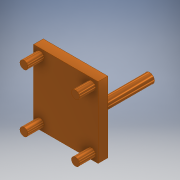
# Autodesk Inventor part: slider
Saved by Autodesk Inventor 2018 (Build 220112000, 112)
## iProperties
Created: 2024-05-02
Part Number: slider
Material: Gold
Document SubType Name: Modeling
Designer: neo
Density: 19.3 g/cm^3
Appearance: Metal 1600F Hot
Author: neo
Autodesk Inventor part; units mm, degrees
ref_plane "YZ Plane" through (0, 0, 0) normal (1, 0, 0) x (0, 1, 0)
ref_plane "XZ Plane" through (0, 0, 0) normal (0, 1, 0) x (-1, 0, 0)
ref_plane "XY Plane" through (0, 0, 0) normal (0, 0, 1) x (1, 0, 0)
sketch "Sketch1" plane through (0, 0, 0) normal (0, 1, 0) x (-1, 0, 0)
  line L0 (15.7413, 3.3999) -> (-17.2771, 3.3999)
  line L1 (0.4016, 18.4289) -> (0.4016, -19.5807)
  line L2 (10.4016, 14.3999) -> (-9.5984, 14.3999)
  line L3 (-9.5984, 14.3999) -> (-9.5984, -7.6001)
  line L4 (-9.5984, -7.6001) -> (10.4016, -7.6001)
  line L5 (10.4016, -7.6001) -> (10.4016, 14.3999)
  circle A0 centre (8.4016, 12.3999) radius 1.25
  circle A1 centre (8.4016, -5.6001) radius 1.25
  circle A2 centre (-7.5984, 12.3999) radius 1.25
  circle A3 centre (-7.5984, -5.6001) radius 1.25
  circle A4 centre (-5.5984, 3.3999) radius 1.5
  point P0 (0, 0)
  dimension "d0" = 2.5
  dimension "d1" = 18
  dimension "d2" = 22
  dimension "d3" = 20
  dimension "d4" = 16
  dimension "d5" = 3
  dimension "d6" = 16
  constraints: 12 end point, 5 centre point, 3 symmetric about line, 2 horizontal, 2 parallel, 1 perpendicular, 1 point on line, 1 vertical, 5 other
  measures "d0" diameter of A0
  measures "d1" distance of A1.centre A0.centre
  measures "d2" distance of L4.end L2.start
  measures "d3" distance of L3.end L4.end
  measures "d4" distance of A2.centre A0.centre
  measures "d5" diameter of A4
  measures "d6" distance from line of L5 A4.centre
extrude "Extrusion1" add sketch "Sketch1" along normal blind 3 contours L5 L4 L1 L0 | L0 L1 L2 L5 | L1 L4 L3 L0 A4 | L0 A4 L3 L2 L1
extrude "Extrusion2" add sketch "Sketch1" along normal blind 20 contours A4 L0 | L0 A4
extrude "Extrusion3" add sketch "Sketch1" against normal blind 5 contours A0 | A1 | A2 | A3
body "Solid1"
